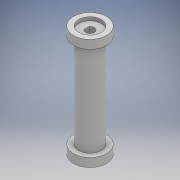
# Autodesk Inventor part: Spool_revB3
Saved by Autodesk Inventor 2017 (Build 210142000, 142)
## iProperties
Created: 2017-04-30
Part Number: Spool_revB3
Material: Generic
Document SubType Name: Modeling
Designer: s4321966
Density: 1 g/cm^3
Appearance: Default
Author: s4321966
Autodesk Inventor part; units mm, degrees
ref_plane "YZ Plane" through (0, 0, 0) normal (1, 0, 0) x (0, 1, 0)
ref_plane "XZ Plane" through (0, 0, 0) normal (0, 1, 0) x (-1, 0, 0)
ref_plane "XY Plane" through (0, 0, 0) normal (0, 0, 1) x (1, 0, 0)
sketch "Sketch1" plane through (0, 0, 0) normal (1, 0, 0) x (0, 1, 0)
  line L0 (0, 0) -> (2.5, 0)
  line L1 (0, 0) -> (4, 0)
  line L2 (2.5, 0) -> (2.5, -7)
  line L3 (2.5, -7) -> (0, -7)
  line L4 (0, -7) -> (20, -7)
  line L5 (4, 0) -> (4, -7)
  line L6 (2.5, -7) -> (2.5, -41)
  line L7 (20, -7) -> (20, -11)
  line L8 (20, -11) -> (2.5, -11)
  line L9 (20, -7) -> (22.5, -7)
  line L10 (22.5, -7) -> (22.5, -11)
  line L11 (22.5, -11) -> (20, -11)
  line L12 (20, -11) -> (20, -7)
  line L13 (20, -7) -> (20, -11)
  line L14 (4, 0) -> (2.5, 0)
  line L15 (2.5, 0) -> (2.5, -11)
  line L16 (2.5, -11) -> (4, -11)
  line L17 (4, -11) -> (4, 0)
  line L18 (2.5, -11) -> (22.5, -11)
  line L19 (22.5, -11) -> (22.5, -7)
  line L20 (22.5, -7) -> (2.5, -7)
  line L21 (2.5, -7) -> (2.5, -11)
  line L22 (2.5, -11) -> (6.5, -11)
  line L23 (0, -7) -> (0, -105.9451)
  line L24 (2.5, -41) -> (25, -41)
  line L25 (0, -82) -> (2.5, -82)
  line L26 (0, -82) -> (4, -82)
  line L27 (2.5, -82) -> (2.5, -75)
  line L28 (2.5, -75) -> (0, -75)
  line L29 (0, -75) -> (20, -75)
  line L30 (4, -82) -> (4, -75)
  line L31 (20, -75) -> (20, -71)
  line L32 (20, -71) -> (2.5, -71)
  line L33 (20, -75) -> (22.5, -75)
  line L34 (22.5, -75) -> (22.5, -71)
  line L35 (22.5, -71) -> (20, -71)
  line L36 (20, -71) -> (20, -75)
  line L37 (20, -75) -> (20, -71)
  line L38 (4, -82) -> (2.5, -82)
  line L39 (2.5, -82) -> (2.5, -71)
  line L40 (2.5, -71) -> (4, -71)
  line L41 (4, -71) -> (4, -82)
  line L42 (2.5, -71) -> (22.5, -71)
  line L43 (22.5, -71) -> (22.5, -75)
  line L44 (22.5, -75) -> (2.5, -75)
  line L45 (2.5, -75) -> (2.5, -71)
  line L46 (2.5, -71) -> (6.5, -71)
  line L47 (2.5, -11) -> (6.5, -11)
  line L48 (6.5, -11) -> (6.5, -71)
  line L49 (6.5, -71) -> (2.5, -71)
  line L50 (2.5, -71) -> (2.5, -11)
  line L51 (6.5, -11) -> (9.5, -11)
  line L52 (9.5, -11) -> (9.5, -14)
  line L53 (9.5, -14) -> (6.5, -14)
  line L54 (6.5, -14) -> (6.5, -11)
  line L55 (6.5, -71) -> (9.5, -71)
  line L56 (9.5, -71) -> (9.5, -68)
  line L57 (9.5, -68) -> (6.5, -68)
  line L58 (6.5, -68) -> (6.5, -71)
  dimension "d1" = 2.5
  dimension "d2" = 4
  dimension "d3" = 7
  dimension "d4" = 20
  dimension "d5" = 34
  dimension "d9" = 4
  dimension "d12" = 2.5
  dimension "d13" = 4
  dimension "d55" = 22.5
  dimension "d56" = 4
  dimension "d80" = 3
  dimension "d81" = 3
  dimension "d82" = 3
  dimension "d83" = 3
  constraints: 118 end point, 17 symmetric about line, 12 parallel, 11 horizontal, 9 perpendicular, 5 point on line, 3 vertical
  measures "d1" distance of L0.start L0.end
  measures "d2" distance of L0.start L1.end
  measures "d3" distance of L0.end L2.end
  measures "d4" distance of L3.end L4.end
  measures "d5" distance of L2.end L6.end
  measures "d9" distance of L4.end L7.end
  measures "d12" distance of L10.end L11.end
  measures "d13" distance of L9.end L10.end
  measures "d55" distance of L6.end L24.end
  measures "d56" distance of L46.end L49.end
  measures "d80" distance of L52.end L53.end
  measures "d81" distance of L51.end L52.end
  measures "d82" distance of L57.end L56.end
  measures "d83" distance of L56.end L55.end
revolve "Revolution2" add sketch "Sketch1" angle 360 about axis through (0, 0, -7) along (0, 0, -1) contours L1 L5 L4 L2 | L4 L17 L8 L6 | L4 L7 L8 L17 | L8 L48 L24 L6 | L9 L10 L11 L7 | L24 L48 L32 L50 | L8 L52 L53 L48 | L29 L30 L26 L27 | L39 L32 L41 L29 | L41 L32 L31 L29 | L57 L56 L32 L48 | L31 L35 L34 L33
sketch "Sketch6" plane through (0, 0, 0) normal (0, 1, 0) x (-1, 0, 0)
  line L0 (-2.5, -82) -> (2.5, -82) projected
  line L1 (0, -82) -> (0, -62)
  line L2 (0, -82) -> (20, -82) construction
  line L3 (0, -65) -> (15, -65) construction
  line L4 (0, -59) -> (15, -59) construction
  line L5 (10.6066, -48.3934) -> (10.6066, -54.3934)
  line L6 (0, -65) -> (0, -59)
  line L7 (0, -62) -> (0, -59.5)
  line L8 (0, -59.5) -> (10.6066, -48.8934)
  line L9 (10.6066, -48.8934) -> (10.6066, -53.8934)
  line L10 (10.6066, -53.8934) -> (0, -64.5)
  line L11 (0, -59.5) -> (0, -64.5)
  point P0 (0, 0)
  dimension "d64" = 20
  dimension "d65" = 90
  dimension "d69" = 15
  dimension "d71" = 15
  dimension "d75" = 2.5
  dimension "d76" = 5
  constraints: 22 end point, 5 point on line, 3 horizontal, 2 vertical, 1 midpoint, 1 parallel, 1 perpendicular
  measures "d64" distance of L1.start L1.end
  measures "d65" angle of L2 L1
  measures "d69" distance of L3.start L5.end
  measures "d71" distance of L4.start L5.start
  measures "d75" distance of L1.end L7.end
  measures "d76" distance of L8.end L9.end
extrude "Extrusion6" cut sketch "Sketch6" along normal mid plane 5
sketch "Sketch7" plane through (0, 0, 0) normal (0, 0, 1) x (1, 0, 0)
  arc A0 (-1.9966, -1.5104) -> (-1.9966, 1.4896) centre (0.0034, -0.0104) ccw
  line L0 (-1.9966, -0.0104) -> (-1.9966, 1.4896)
  line L1 (-1.9966, -0.0104) -> (-1.9966, -1.5104)
  line L2 (-1.9966, 1.4896) -> (-1.9966, -2.007)
  line L3 (-1.9966, -2.007) -> (-3.9862, -2.007)
  line L4 (-3.9862, -2.007) -> (-3.9862, 1.4896)
  line L5 (-3.9862, 1.4896) -> (-1.9966, 1.4896)
  line L6 (-1.9966, -1.5104) -> (-3.2272, -1.5104)
  line L7 (-3.2272, -1.5104) -> (-3.2272, 1.4896)
  line L8 (-3.2272, 1.4896) -> (-1.9966, 1.4896)
  line L9 (-1.9966, 1.4896) -> (-1.9966, -1.5104)
  point P0 (0, 0)
  point P1 (0, 0)
  dimension "d77" = 5
  constraints: 20 end point, 4 parallel, 2 perpendicular, 2 point on circle, 2 point on line, 1 centre point, 1 horizontal
  measures "d77" diameter of A0
extrude "Extrusion7" add sketch "Sketch7" against normal blind 26 contours L6 L7 L5 L0 L1
sketch "Sketch11" plane through (0, 0, -71) normal (0, 0, 1) x (1, 0, 0)
  circle A0 centre (0, 0) radius 2.5 projected
  circle A1 centre (0, 0) radius 9.5
  arc A2 (0, 2.5) -> (0, -2.5) centre (0, 0) ccw projected
  circle A3 centre (0, 0) radius 46.837
  point P0 (0, 0)
  dimension "d90" = 19
  constraints: 2 centre point, 2 coincident
  measures "d90" diameter of A1
extrude "Extrusion11" cut sketch "Sketch11" against normal blind 100 contours A0 | A1 | A3
sketch "Sketch12" plane through (0, 0, -71) normal (0, 0, -1) x (-1, 0, 0)
  circle A0 centre (0, 0) radius 9.5 projected
  circle A1 centre (0, 0) radius 9.5
  circle A2 centre (0, 0) radius 6.5
  point P0 (0, 0)
  constraints: 2 centre point, 2 coincident
extrude "Extrusion12" add sketch "Sketch12" along normal blind 2
sketch "Sketch13" plane through (0, 0, -11) normal (0, 0, -1) x (-1, 0, 0)
  circle A0 centre (0, 0) radius 46.586
  constraints: 1 centre point, 1 coincident
extrude "Extrusion13" cut sketch "Sketch13" against normal blind 30
sketch "Sketch14" plane through (0, 0, -11) normal (0, 0, 1) x (1, 0, 0)
  circle A0 centre (0, 0) radius 9.5
  circle A1 centre (0, 0) radius 9.5
  arc A2 (0, 2.5) -> (0, -2.5) centre (0, 0) ccw projected
  circle A3 centre (0, 0) radius 6.5
  dimension "d97" = 19
  dimension "d98" = 13
  constraints: 3 centre point, 3 coincident
  measures "d97" diameter of A1
  measures "d98" diameter of A3
extrude "Extrusion14" add sketch "Sketch14" along normal blind 2
body "Solid2"
